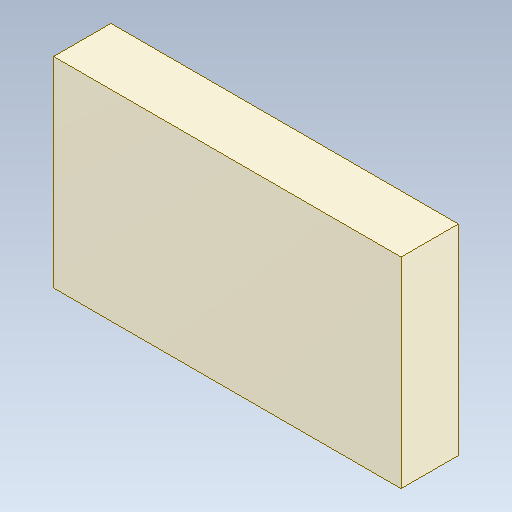
# Autodesk Inventor part: MOMENTARY-SWITCH-SPST-SMD-6_0X3_5MM
Saved by Autodesk Inventor 2020 (Build 240168000, 168)
## iProperties
Created: 2019-05-24
Part Number: MOMENTARY-SWITCH-SPST-SMD-6_0X3_5MM
Material: Generic
Document SubType Name: Modeling
Designer: psrob
Density: 1 g/cm^3
Appearance: TACTILE_SWITCH_SMD_6_0X3_5MM, MOMENTARY-SWITCH-SPST-SMD-6_0X3_5MM
Author: psrob
Autodesk Inventor part; units mm, degrees
ref_plane "YZ Plane" through (0, 0, 0) normal (1, 0, 0) x (0, 1, 0)
ref_plane "XZ Plane" through (0, 0, 0) normal (0, 1, 0) x (-1, 0, 0)
ref_plane "XY Plane" through (0, 0, 0) normal (0, 0, 1) x (1, 0, 0)
sketch3d "TACTILE_SWITCH_SMD_6_0X3_5MM, MOMENTARY-SWITCH-SPST-SMD-6_0X"
  constraints: 8 end point
sketch "TACTILE_SWITCH_SMD_6_0X3_5MM, MOMENTARY-SWITCH-SPST-SMD-6_0X3_5MM_54" plane through (0, 0, 0) normal (0, 0, 1) x (1, 0, 0)
  line L0 (-3.0635, 1.75) -> (3, 1.75)
  line L1 (3, 1.75) -> (3, -1.75)
  line L2 (3, -1.75) -> (-3.0635, -1.75)
  line L3 (-3.0635, -1.75) -> (-3.0635, 1.75)
extrude "Extrusion1" add sketch "TACTILE_SWITCH_SMD_6_0X3_5MM, MOMENTARY-SWITCH-SPST-SMD-6_0X3_5MM_54" along normal blind 1
body "Solid1"
